Autodesk Inventor part; units mm, degrees
(part 2 of 2)
sketch "Sketch4" plane through (0, 0, 0) normal (-1, 0, 0) x (0, 0, 1)
  circle A0 centre (-20.465, 2.3012) radius 45
  line L0 (40.535, 4.2654) -> (40.535, -113.663) projected
  line L1 (40.535, -54.6988) -> (-74.4653, -54.6988) construction
  line L2 (-74.4653, -113.663) -> (-74.4653, 4.2654) projected
  circle A1 centre (-20.465, 2.3012) radius 43
  line L3 (-20.465, 2.3012) -> (24.535, 2.3012)
  line L4 (-20.465, 2.3012) -> (18.5062, -20.1988)
  line L5 (-20.465, 2.3012) -> (2.035, 41.2723)
  line L6 (-20.465, 2.3012) -> (18.5062, 24.8012)
  line L7 (-20.465, 2.3012) -> (-42.965, 41.2723)
  line L8 (-20.465, 2.3012) -> (-20.465, 47.3012)
  line L9 (-20.465, 2.3012) -> (-65.465, 2.3012)
  line L10 (-20.465, 2.3012) -> (-59.4361, 24.8012)
  line L11 (-20.465, 2.3012) -> (-42.965, -36.6699)
  line L12 (-20.465, 2.3012) -> (-59.4361, -20.1988)
  line L13 (-20.465, 2.3012) -> (2.035, -36.6699)
  line L14 (-20.465, 2.3012) -> (-20.465, -42.6988)
  circle A2 centre (-20.465, -111.6988) radius 45
  line L15 (-74.4653, 4.2654) -> (-74.4653, -113.663)
  circle A3 centre (-20.465, -111.6988) radius 43
  line L16 (-20.465, -111.6988) -> (24.535, -111.6988)
  line L17 (-20.465, -111.6988) -> (18.5062, -89.1988)
  line L18 (-20.465, -111.6988) -> (2.035, -150.6699)
  line L19 (-20.465, -111.6988) -> (18.5062, -134.1988)
  line L20 (-20.465, -111.6988) -> (-42.965, -150.6699)
  line L21 (-20.465, -111.6988) -> (-20.465, -156.6988)
  line L22 (-20.465, -111.6988) -> (-65.465, -111.6988)
  line L23 (-20.465, -111.6988) -> (-59.4361, -134.1988)
  line L24 (-20.465, -111.6988) -> (-42.965, -72.7277)
  line L25 (-20.465, -111.6988) -> (-59.4361, -89.1988)
  line L26 (-20.465, -111.6988) -> (2.035, -72.7277)
  line L27 (-20.465, -111.6988) -> (-20.465, -66.6988)
  circle A4 centre (12.535, -54.6988) radius 10
  line L28 (40.535, 4.2654) -> (40.535, -113.663) projected
  circle A5 centre (12.535, -54.6988) radius 8
  line L29 (12.535, -54.6988) -> (22.535, -54.6988)
  line L30 (12.535, -54.6988) -> (21.1953, -59.6988)
  line L31 (12.535, -54.6988) -> (21.1953, -49.6988)
  line L32 (12.535, -54.6988) -> (17.535, -46.0385)
  line L33 (12.535, -54.6988) -> (12.535, -44.6988)
  line L34 (12.535, -54.6988) -> (7.535, -46.0385)
  line L35 (12.535, -54.6988) -> (3.8748, -49.6988)
  line L36 (12.535, -54.6988) -> (2.535, -54.6988)
  line L37 (12.535, -54.6988) -> (3.8748, -59.6988)
  line L38 (12.535, -54.6988) -> (7.535, -63.3591)
  line L39 (12.535, -54.6988) -> (12.535, -64.6988)
  line L40 (12.535, -54.6988) -> (17.535, -63.3591)
  line L41 (-55.465, -54.6988) -> (-46.8047, -59.6988)
  line L42 (-55.465, -54.6988) -> (-45.465, -54.6988)
  line L43 (-55.465, -54.6988) -> (-46.8047, -49.6988)
  line L44 (-55.465, -54.6988) -> (-50.465, -46.0385)
  line L45 (-55.465, -54.6988) -> (-55.465, -44.6988)
  line L46 (-55.465, -54.6988) -> (-55.465, -64.6988)
  line L47 (-55.465, -54.6988) -> (-50.465, -63.3591)
  line L48 (-55.465, -54.6988) -> (-60.465, -46.0385)
  circle A6 centre (-55.465, -54.6988) radius 10
  circle A7 centre (-55.465, -54.6988) radius 8
  line L49 (-55.465, -54.6988) -> (-60.465, -63.3591)
  line L50 (-55.465, -54.6988) -> (-64.1252, -49.6988)
  line L51 (-55.465, -54.6988) -> (-64.1252, -59.6988)
  line L52 (-55.465, -54.6988) -> (-65.465, -54.6988)
  point P0 (0, 0)
  point P1 (0, -109.3976)
  point P2 (-41.965, -148.9379)
  point P3 (-20.465, -154.6988)
  point P4 (16.7741, -133.1988)
  point P5 (1.035, -148.9379)
  point P6 (16.7741, -90.1988)
  point P7 (22.535, -111.6988)
  point P8 (-20.465, -68.6988)
  point P9 (1.035, -74.4597)
  point P10 (2.035, -72.7277)
  point P11 (-57.7041, -90.1988)
  point P12 (-41.965, -74.4597)
  point P13 (-57.7041, -133.1988)
  point P14 (-63.465, -111.6988)
  point P15 (-20.465, 45.3012)
  point P16 (1.035, 39.5403)
  point P17 (-57.7041, 23.8012)
  point P18 (-41.965, 39.5403)
  point P19 (-57.7041, -19.1988)
  point P20 (-63.465, 2.3012)
  point P21 (-20.465, -40.6988)
  point P22 (-41.965, -34.9379)
  point P23 (1.035, -34.9379)
  point P24 (2.035, -36.6699)
  point P25 (16.7741, -19.1988)
  point P26 (16.7741, 23.8012)
  point P27 (22.535, 2.3012)
  point P28 (-55.465, -46.6988)
  point P29 (-51.465, -47.7706)
  point P30 (-62.3932, -50.6988)
  point P31 (-59.465, -47.7706)
  point P32 (-63.465, -54.6988)
  point P33 (-62.3932, -58.6988)
  point P34 (-59.465, -61.627)
  point P35 (-55.465, -62.6988)
  point P36 (-48.5368, -58.6988)
  point P37 (-51.465, -61.627)
  point P38 (-48.5368, -50.6988)
  point P39 (-47.465, -54.6988)
  point P40 (12.535, -46.6988)
  point P41 (16.535, -47.7706)
  point P42 (5.6068, -50.6988)
  point P43 (8.535, -47.7706)
  point P44 (5.6068, -58.6988)
  point P45 (4.535, -54.6988)
  point P46 (12.535, -62.6988)
  point P47 (8.535, -61.627)
  point P48 (16.535, -61.627)
  point P49 (19.4632, -58.6988)
  point P50 (19.4632, -50.6988)
  point P51 (20.535, -54.6988)
  dimension "d50" = 90
  dimension "d51" = 57
  dimension "d52" = 61
  dimension "d53" = 2
  dimension "d54" = 30
  dimension "d57" = 360
  dimension "d61" = 20
  dimension "d62" = 28
  dimension "d63" = 2
  dimension "d64" = 30
  dimension "d67" = 360
  dimension "d71" = 68
  constraints: 100 end point, 21 symmetric about line, 8 centre point, 8 point on circle, 4 coincident, 3 midpoint, 2 horizontal, 2 point on line, 92 other
  measures "d50" diameter of A0
  measures "d51" distance from line of L1 L3.start
  measures "d52" distance from line of L3.start L0
  measures "d53" radial gap between concentric circles of A0 A1
  measures "d54" angle of L4 L3
  measures "d61" diameter of A4
  measures "d62" distance of point (40.535, -54.699) L29.start
  measures "d63" radial gap between concentric circles of A4 A5
  measures "d64" angle of L30 L1
  measures "d71" distance of L29.start L41.start
extrude "Extrusion24" cut sketch "Sketch4" against normal through all contours L3 A1 L6 A0 | A0 L13 A1 L4 | L5 A1 L8 A0 | A0 L11 A1 L14 | A1 L10 A0 L7 | A1 L12 A0 L9 | L16 A3 L17 A2 | A2 L18 A3 L19 | L26 A3 L27 A2 | A2 L20 A3 L21 | A3 L23 A2 L22 | A3 L25 A2 L24 | L29 A5 L31 A4 | A4 L40 A5 L30 | L32 A5 L33 A4 | A4 L38 A5 L39 | A5 L35 A4 L34 | A5 L37 A4 L36 | L41 A6 L47 A7 | A7 L43 A6 L42 | A7 L45 A6 L44 | L46 A6 L49 A7 | A7 L50 A6 L48 | L51 A6 L52 A7
body "Solid4"
